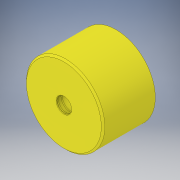
# Autodesk Inventor part: support_entree_air
Saved by Autodesk Inventor 2019 (Build 230136000, 136)
## iProperties
Created: 2018-05-05
Part Number: support_entree_air
Material: Générique
Document SubType Name: Modeling
Designer: Theo
Density: 1 g/cm^3
Appearance: Jaune canari
Author: Theo
Autodesk Inventor part; units mm, degrees
ref_plane "YZ Plane" through (0, 0, 0) normal (1, 0, 0) x (0, 1, 0)
ref_plane "XZ Plane" through (0, 0, 0) normal (0, 1, 0) x (-1, 0, 0)
ref_plane "XY Plane" through (0, 0, 0) normal (0, 0, 1) x (1, 0, 0)
sketch "Esquisse1" plane through (0, 0, 0) normal (1, 0, 0) x (0, 1, 0)
  line L0 (0, 0) -> (0, -64.1706)
  line L1 (22.5, -1) -> (22.5, -30)
  line L2 (22.5, -1) -> (21.5, 0)
  line L3 (21.5, 0) -> (4.5, 0)
  arc A0 (4.5, 0) -> (4.25, -0.25) centre (4.5, -0.25) ccw
  line L4 (4.25, -0.25) -> (4.25, -0.5)
  arc A1 (4.25, -0.5) -> (4.4102, -1.3241) centre (6.45, -0.5) ccw
  line L5 (4, -0.25) -> (4, -0.5) construction
  line L6 (4.4102, -1.3241) -> (5.3398, -3.625)
  arc A2 (5.5, -4.4491) -> (5.3398, -3.625) centre (3.3, -4.4491) ccw
  line L7 (5.5, -4.4491) -> (5.5, -14)
  line L8 (5.25, -4.4491) -> (5.25, -14) construction
  arc A3 (5.5, -14) -> (5.8514, -14.7611) centre (6.4999, -14) ccw
  line L9 (22.5, -30) -> (19.5, -30)
  line L10 (19.5, -30) -> (18.5, -29)
  line L11 (18.5, -29) -> (18.5, -26)
  line L12 (18.1486, -25.2388) -> (5.8514, -14.7611)
  arc A4 (18.5, -26) -> (18.1486, -25.2388) centre (17.5, -26) ccw
  dimension "d0" = 45
  dimension "d1" = 1
  dimension "d2" = 1
  dimension "d3" = 0.25
  dimension "d4" = 2.2
  dimension "d5" = 0.5
  dimension "d6" = 0.25
  dimension "d7" = 8
  dimension "d8" = 0.25
  dimension "d9" = 10.5
  dimension "d10" = 158
  dimension "d11" = 0.9999
  dimension "d12" = 1
  dimension "d13" = 1
  dimension "d14" = 4
  dimension "d15" = 1
  dimension "d16" = 30
  dimension "d17" = 14
  dimension "d20" = 4
  constraints: 26 end point, 10 point on circle, 10 tangent, 7 vertical, 5 centre point, 5 horizontal alignment, 2 horizontal, 1 equal radius
  measures "d0" diameter of L1 L0
  measures "d1" horizontal distance of L1.start L2.end
  measures "d2" horizontal distance of L1.start L2.end
  measures "d3" radius of A0
  measures "d4" radius of A1
  measures "d5" vertical distance of L4.end L3.end
  measures "d6" distance between parallel lines of L4 L5
  measures "d7" diameter of L5 L0
  measures "d8" distance between parallel lines of L7 L8
  measures "d9" diameter of L8 L0
  measures "d10" angle of L7 L6
  measures "d11" radius of A3
  measures "d12" horizontal distance of L9.end L10.end
  measures "d13" horizontal distance of L9.end L10.end
  measures "d14" distance between parallel lines of L1 L11
  measures "d15" radius of A4
  measures "d16" distance between parallel lines of L3 L9
  measures "d17" distance from line of L7.end L3
  measures "d20" vertical distance of L11.end L9.end
revolve "Révolution1" add sketch "Esquisse1" angle 360 about axis through (0, 0, 0) along (0, 0, -1)
equation "\"d2\" = d1"
equation "\"d13\" = d12"
